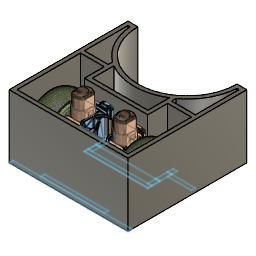
MiniSoccer (Autodesk Fusion 360 design; units mm, degrees)
part number: 2025-12-04-09-52-39-113
Autodesk Fusion 360 part; units mm, degrees
sketch "Sketch1" plane through (0, 0, 0) normal (0, 0, 1) x (1, 0, 0)
  line L0 (0, 0) -> (150, 0)
  line L1 (150, 0) -> (150, -150)
  line L2 (150, -150) -> (0, -150)
  line L3 (0, -150) -> (0, 0)
  line L4 (0, -150) -> (60, -150)
  line L5 (60, -150) -> (60, 0)
  line L6 (60, 0) -> (0, 0)
  line L7 (0, 0) -> (0, -150)
  line L8 (150, -150) -> (90, -150)
  line L9 (90, -150) -> (90, 0)
  line L10 (90, 0) -> (150, 0)
  line L11 (150, 0) -> (150, -150)
  line L12 (0, -150) -> (150, -150)
  line L13 (150, -150) -> (150, -70)
  line L14 (150, -70) -> (0, -70)
  line L15 (0, -70) -> (0, -150)
  line L16 (0, -75) -> (150, -75)
  line L17 (75, -150) -> (75, 0)
  line L18 (75, -70) -> (73.1201, -70)
  line L19 (75, 0) -> (75, -35)
  line L20 (125, -70) -> (25, -70)
  line L21 (25, -70) -> (25, 0)
  line L22 (25, 0) -> (125, 0)
  line L23 (125, 0) -> (125, -70)
  line L24 (35, -70) -> (115, -70)
  line L25 (115, -70) -> (115, -150)
  line L26 (115, -150) -> (35, -150)
  line L27 (35, -150) -> (35, -70)
  line L28 (55, -150) -> (55, -70)
  line L29 (95, -150) -> (95, -70)
  arc A0 (5, 0) -> (145, 0) centre (75, 0) ccw
  line L30 (5, 0) -> (5, -70)
  line L31 (145, 0) -> (145, -3.358)
  line L32 (145, -3.358) -> (145, -70)
  arc A1 (15, 0) -> (135, 0) centre (75, 0) ccw
  arc A2 (10, 0) -> (140, 0) centre (75, 0) ccw
  line L33 (35, -70) -> (35, -44.7214)
  line L34 (115, -70) -> (115, -44.7214)
  line L35 (150, -150) -> (146, -150)
  line L36 (146, -150) -> (146, -75)
  line L37 (146, -75) -> (150, -75)
  line L38 (150, -75) -> (150, -150)
  line L39 (0, -75) -> (4, -75)
  line L40 (4, -75) -> (4, -150)
  line L41 (4, -150) -> (0, -150)
  line L42 (0, -150) -> (0, -75)
  line L43 (150, -150) -> (0, -150)
  line L44 (0, -150) -> (0, -146)
  line L45 (0, -146) -> (150, -146)
  line L46 (150, -146) -> (150, -150)
  line L47 (150, 0) -> (0, 0)
  line L48 (0, 0) -> (0, -5)
  line L49 (0, -5) -> (150, -5)
  line L50 (150, -5) -> (150, 0)
  line L51 (130, -5) -> (145, -5)
  line L52 (145, -5) -> (145, -25)
  line L53 (145, -25) -> (130, -25)
  line L54 (130, -25) -> (130, -5)
  line L55 (20, -5) -> (5, -5)
  line L56 (5, -5) -> (5, -25)
  line L57 (5, -25) -> (20, -25)
  line L58 (20, -25) -> (20, -5)
  point P0 (75, -35)
  dimension "d1" = 150
  dimension "d2" = 150
  dimension "d3" = 60
  dimension "d4" = 150
  dimension "d5" = 60
  dimension "d6" = 80
  dimension "d7" = 100
  dimension "d8" = 70
  constraint horizontal L0
  constraint vertical L1
  constraint horizontal L2
  constraint vertical L3
  constraint coincident L0.start L3.end
  constraint horizontal L4
  constraint vertical L5
  constraint horizontal L6
  constraint vertical L7
  constraint horizontal L8
  constraint vertical L9
  constraint horizontal L10
  constraint vertical L11
  constraint horizontal L12
  constraint vertical L13
  constraint horizontal L14
  constraint vertical L15
  constraint midpoint L3 L16.start
  constraint midpoint L1 L16.end
  constraint midpoint L12 L17.start
  constraint midpoint L0 L17.end
  constraint perpendicular L0 L17
  constraint midpoint L14 L18.start
  constraint coincident L14 L18.end
  constraint coincident L17 P0
  constraint horizontal L20
  constraint perpendicular L20 L21
  constraint parallel L20 L22
  constraint parallel L21 L23
  constraint coincident P0 L19.end
  constraint horizontal L24
  constraint vertical L25
  constraint horizontal L26
  constraint vertical L27
  constraint coincident L8 L25.end
  constraint coincident L14 L24.start
  constraint coincident L4 L28.start
  constraint coincident L14 L28.end
  constraint coincident L24 L29.end
  constraint coincident L17.end L19.start
  constraint coincident L18.start A0
  constraint coincident L0 A0.end
  constraint coincident L0 A0.start
  constraint coincident L14 L30.end
  constraint tangent A0 L30
  constraint tangent A0 L31
  constraint coincident L14 L32.end
  constraint perpendicular L14 L32
  constraint coincident L0 A1.end
  constraint coincident L0 A1.start
  constraint coincident L0 A2.end
  constraint coincident L0 A2.start
  constraint coincident A1 L33.end
  constraint perpendicular L24 L33
  constraint coincident A1 L34.end
  constraint perpendicular L24 L34
  constraint horizontal L35
  constraint vertical L36
  constraint horizontal L37
  constraint vertical L38
  constraint coincident L16 L36.end
  constraint horizontal L39
  constraint vertical L40
  constraint horizontal L41
  constraint vertical L42
  constraint coincident L12 L40.end
  constraint horizontal L43
  constraint vertical L44
  constraint horizontal L45
  constraint vertical L46
  constraint coincident L42 L44.end
  constraint horizontal L47
  constraint vertical L48
  constraint horizontal L49
  constraint vertical L50
  constraint coincident L7 L48.end
  constraint horizontal L51
  constraint vertical L52
  constraint horizontal L53
  constraint vertical L54
  constraint coincident L32 L52.end
  constraint coincident L49 L51.start
  constraint horizontal L55
  constraint vertical L56
  constraint horizontal L57
  constraint vertical L58
  constraint coincident L30 L56.end
  constraint coincident L49 L55.start
  measures "d1" distance of L0.start L0.end
  measures "d2" distance of L0.start L2.end
  measures "d3" distance of L2.end L4.end
  measures "d4" distance of L2.end L0.start
  measures "d5" distance of L1.end L8.end
  measures "d6" distance of L2.end L14.end
  measures "d7" distance of L21.end L22.end
  measures "d8" distance of L20.end L21.end
other "Base Mesh Feature1"
other "Base Mesh Feature2"
other "Modify1"
other "Modify2"
other "Modify3"
other "Modify4"
other "Modify5"
other "Modify6"
other "Modify7"
other "Modify8"
other "Modify9"
other "Modify10"
other "CopyPasteMeshes1"
other "CopyPasteMeshes2"
other "Modify11"
other "Modify12"
other "Modify13"
extrude "Extrude14" cut sketch "Sketch1" along normal blind 60 contours A0 L30 L49 L55 | A0 L30 L49 L55 L56 L57 | L14 L21 A0 L30 L57 | L14 L20 L21 A0 L33 | L5 L14 L20 L24 A0 L33 | L9 L14 L20 L24 A0 L34 | L14 L20 L23 A0 L34 | L14 L23 A0 L32 L53 | A0 L31 L32 L49 L51 | A0 L32 L49 L51 L52 L53
extrude "Extrude16" cut sketch "Sketch1" along normal blind 60 contours L0 L6 A0 A2 L47 L49 L55 | A0 A2 L49 L55 L57 | L21 A0 A2 L57 | L0 L10 A0 A2 L47 L49 L51 | L23 A0 A2 L53 | A0 A2 L49 L51 L53
extrude "Extrude17" cut sketch "Sketch1" along normal blind 60 contours L5 L14 L18 L20 L24 A0 | L5 L17 A0 A2 | L9 L14 L20 L24 A0 | L9 L17 A0 A2
sketch "Sketch2" plane through (0, 0, 0) normal (0, 0, 1) x (1, 0, 0)
  line L0 (150, 0) -> (150, -150)
  line L1 (150, -150) -> (0, -150)
  line L2 (0, -150) -> (0, 0)
  line L3 (0, -75) -> (150, -75)
  line L4 (145, -145) -> (5, -145)
  line L5 (5, -145) -> (5, -5)
  line L6 (145, -5) -> (145, -145)
  line L7 (35, -150) -> (60, -150)
  line L8 (90, -150) -> (115, -150)
  line L9 (90, -50) -> (90, -150)
  line L10 (35, -145) -> (5, -145)
  line L11 (5, -145) -> (5, -65)
  line L12 (5, -65) -> (35, -65)
  line L13 (35, -65) -> (35, -145)
  line L14 (145, -145) -> (115, -145)
  line L15 (115, -145) -> (115, -65)
  line L16 (115, -65) -> (145, -65)
  line L17 (145, -65) -> (145, -145)
  line L18 (5, -105) -> (35, -105)
  line L19 (115, -105) -> (145, -105)
  line L20 (130, -65) -> (130, -145)
  line L21 (20, -65) -> (20, -145)
  arc A0 (12.5, 0) -> (137.5, 0) centre (75, 0) ccw
  line L22 (137.5, -50) -> (12.5, -50)
  line L23 (12.5, -50) -> (12.5, 0)
  line L24 (137.5, 0) -> (137.5, -50)
  arc A1 (7.5, 0) -> (142.5, 0) centre (75, 0) ccw
  line L25 (0, 0) -> (12.5, 0)
  line L26 (5, -5) -> (12.7003, -5)
  line L27 (35, -48.0234) -> (35, -150)
  line L28 (60, -150) -> (60, -50)
  line L29 (75, -50) -> (75, -150)
  line L30 (137.5, -50) -> (123.8043, -39.0434) construction
  line L31 (115, -150) -> (115, -48.0234)
  line L32 (115, -5) -> (115, 0)
  line L33 (137.2997, -5) -> (145, -5)
  line L34 (137.5, 0) -> (150, 0)
  line L35 (14.1146, -14.1146) -> (5, -5) construction
  line L36 (12.5, -50) -> (26.1957, -39.0434) construction
  line L37 (145, -145) -> (50, -50) construction
  line L38 (5, -145) -> (75, -75) construction
  line L39 (82.9725, -67.0275) -> (100, -50) construction
  line L40 (135.8854, -14.1146) -> (145, -5) construction
  point P0 (75, 0)
  dimension "d55" = 125
  constraint horizontal L25
  constraint vertical L0
  constraint horizontal L1
  constraint vertical L2
  constraint coincident L2.end L25.start
  constraint midpoint L2 L3.start
  constraint midpoint L0 L3.end
  constraint midpoint L1 L29.end
  constraint horizontal L4
  constraint perpendicular L4 L5
  constraint parallel L4 L26
  constraint parallel L5 L6
  constraint coincident L38.end L37
  constraint midpoint L3 L38.end
  constraint horizontal L7
  constraint vertical L28
  constraint coincident L1 L7.start
  constraint horizontal L8
  constraint vertical L31
  constraint vertical L9
  constraint coincident L32.end L25
  constraint coincident L1 L8.start
  constraint horizontal L10
  constraint vertical L11
  constraint horizontal L12
  constraint vertical L13
  constraint coincident L5 L11.end
  constraint coincident L4 L10.start
  constraint horizontal L14
  constraint vertical L15
  constraint horizontal L16
  constraint vertical L17
  constraint coincident L15.end L31
  constraint midpoint L11 L18.start
  constraint midpoint L13 L18.end
  constraint midpoint L15 L19.start
  constraint midpoint L17 L19.end
  constraint midpoint L16 L20.start
  constraint midpoint L14 L20.end
  constraint midpoint L12 L21.start
  constraint midpoint L10 L21.end
  constraint coincident A0.end L25
  constraint horizontal L22
  constraint perpendicular L22 L23
  constraint coincident P0 L30
  constraint coincident P0 L36
  constraint coincident A1.start L25
  constraint coincident A1.end L25
  constraint coincident A0 L26.end
  constraint coincident L22 L29.start
  constraint collinear L31 L32
  constraint coincident A0 L33.start
  constraint coincident L22 L28.end
  constraint coincident L22 L9.start
  constraint coincident A0 L35.start
  constraint collinear L35 L37
  constraint coincident A0 L36.end
  constraint coincident L22 L37.end
  constraint coincident A0 L27.start
  constraint coincident A1 L39.start
  constraint collinear L38 L39
  constraint coincident L22 L39.end
  constraint coincident A0 L40.start
  constraint coincident A0 L31.end
  constraint coincident A0 L30.end
  measures "d55" diameter of A0
other "Modify14"
other "Modify15"
extrude "Extrude24" add sketch "Sketch2" along normal blind 80 separate body contours L0 L3 L6 L17 A1 L33 L34 | L0 L1 L3 L4 L6 L14 L17 L31 | L24 A1 L33 L34 | L1 L4 L8 L9 L31 | L1 L4 L9 L29 | L1 L4 L28 L29 | L1 L4 L7 L27 L28 | L1 L2 L3 L4 L5 L10 L11 L27 | L2 L3 L5 L11 A1 L25 L26 | L23 A1 L25 L26 makes body 1
other "Modify16"
other "Modify17"
other "Modify18"
other "Modify19"
other "CopyPasteMeshes3"
other "Modify20"
other "Modify21"
extrude "Extrude25" add sketch "Sketch2" along normal blind 80 contours L24 A1 L33 | A0 L22 L24 A1 L31 L33 | L22 A1 L31 | A0 L22 L31 | L9 A0 L22 A1 L31 | L9 A0 A1 L29 | A0 A1 L28 L29 | A0 L22 A1 L27 L28 | L22 A1 L27 | A0 L22 L27 | A0 L22 L23 A1 L26 L27 | L23 A1 L26 bodies 1
other "Base Mesh Feature3"
other "Modify22"
other "Modify23"
other "Modify24"
other "Modify25"
other "Modify26"
other "Modify27"
sketch "Sketch3" plane through (0, 0, 0) normal (0, 0, 1) x (1, 0, 0)
  line L0 (35, -75) -> (115, -75)
  line L1 (115, -75) -> (115, -90)
  line L2 (115, -90) -> (35, -90)
  line L3 (35, -90) -> (35, -75)
  line L4 (35, -90) -> (115, -90)
  line L5 (115, -90) -> (115, -85)
  line L6 (115, -85) -> (35, -85)
  line L7 (35, -85) -> (35, -90)
  line L8 (35, -145) -> (115, -145)
  line L9 (115, -145) -> (115, -140)
  line L10 (115, -140) -> (35, -140)
  line L11 (35, -140) -> (35, -145)
  line L12 (0, -145) -> (150, -145)
  line L13 (150, -145) -> (150, -150)
  line L14 (150, -150) -> (0, -150)
  line L15 (0, -150) -> (0, -145)
  line L16 (110, -75) -> (115, -75)
  line L17 (115, -75) -> (115, -60)
  line L18 (115, -60) -> (110, -60)
  line L19 (110, -60) -> (110, -75)
  line L20 (145, -65) -> (115, -65)
  line L21 (115, -65) -> (115, -60)
  line L22 (115, -60) -> (145, -60)
  line L23 (145, -60) -> (145, -65)
  line L24 (35, -75) -> (40, -75)
  line L25 (40, -75) -> (40, -60)
  line L26 (40, -60) -> (35, -60)
  line L27 (35, -60) -> (35, -75)
  line L28 (35, -60) -> (5, -60)
  line L29 (5, -60) -> (5, -65)
  line L30 (5, -65) -> (35, -65)
  line L31 (35, -65) -> (35, -60)
  line L32 (35, -60) -> (40, -60)
  line L33 (40, -60) -> (40, -54.3331)
  line L34 (40, -54.3331) -> (35, -54.3331)
  line L35 (35, -54.3331) -> (35, -60)
  line L36 (110, -60) -> (115, -60)
  line L37 (115, -60) -> (115, -53.1436)
  line L38 (115, -53.1436) -> (110, -53.1436)
  line L39 (110, -53.1436) -> (110, -60)
  line L40 (35, -75) -> (40, -75)
  line L41 (40, -75) -> (40, -85)
  line L42 (40, -85) -> (35, -85)
  line L43 (35, -85) -> (35, -75)
  line L44 (110, -75) -> (115, -75)
  line L45 (115, -75) -> (115, -85)
  line L46 (115, -85) -> (110, -85)
  line L47 (110, -85) -> (110, -75)
  constraint horizontal L0
  constraint vertical L1
  constraint horizontal L2
  constraint vertical L3
  constraint horizontal L4
  constraint vertical L5
  constraint horizontal L6
  constraint vertical L7
  constraint coincident L1 L5.end
  constraint horizontal L8
  constraint vertical L9
  constraint horizontal L10
  constraint vertical L11
  constraint horizontal L12
  constraint vertical L13
  constraint horizontal L14
  constraint vertical L15
  constraint horizontal L16
  constraint vertical L17
  constraint horizontal L18
  constraint vertical L19
  constraint coincident L0 L16.start
  constraint horizontal L20
  constraint vertical L21
  constraint horizontal L22
  constraint vertical L23
  constraint horizontal L24
  constraint vertical L25
  constraint horizontal L26
  constraint vertical L27
  constraint horizontal L28
  constraint vertical L29
  constraint horizontal L30
  constraint vertical L31
  constraint horizontal L32
  constraint vertical L33
  constraint horizontal L34
  constraint vertical L35
  constraint horizontal L36
  constraint vertical L37
  constraint horizontal L38
  constraint vertical L39
  constraint horizontal L40
  constraint vertical L41
  constraint horizontal L42
  constraint vertical L43
  constraint coincident L6 L41.end
  constraint horizontal L44
  constraint vertical L45
  constraint horizontal L46
  constraint vertical L47
extrude "Extrude26" add sketch "Sketch3" along normal blind 80 separate body contours L1 L2 L3 L4 L5 L6 L7 L42 L46 makes body 2
extrude "Extrude27" add sketch "Sketch2" along normal blind 5 contours L3 L4 L9 L15 L31 | L3 L4 L9 L29 | L3 L4 L28 L29 | L3 L4 L13 L27 L28 bodies 2
extrude "Extrude28" add sketch "Sketch2" along normal blind 5 contours L6 L16 L22 L24 A1 L31 L33 | L22 L24 A1 | L3 L9 L15 A1 L31 | L3 L9 A1 L29 | L3 A1 L28 L29 | L3 L13 A1 L27 L28 | L5 L12 L22 L23 A1 L26 L27 | L22 L23 A1 bodies 1 2
extrude "Extrude29" cut sketch "Sketch3" along normal blind 80 contours L8 L12 L13 L14 L15 bodies 1
extrude "Extrude30" add sketch "Sketch3" along normal blind 80 contours L0 L24 L25 L26 L27 L31 L32 L40 | L27 L28 L29 L30 L31 | L0 L16 L17 L18 L19 L21 L36 L44 | L17 L20 L21 L22 L23 bodies 1
extrude "Extrude31" add sketch "Sketch2" along normal blind 80 contours A0 L24 L33 bodies 1
extrude "Extrude32" add sketch "Sketch2" along normal blind 80 contours A0 L23 L26 bodies 1
other "Base Mesh Feature4"
other "Modify28"
other "Modify29"
extrude "Extrude33" add sketch "Sketch3" along normal blind 80 contours L8 L12 L13 L14 L15 bodies 1
extrude "Extrude34" cut sketch "Sketch2" along normal blind 5 contours L6 L16 L22 L24 A1 L31 L33 | L22 L24 A1 | L5 L12 L22 L23 A1 L26 L27 | L22 L23 A1 bodies 1
extrude "Extrude35" add sketch "Sketch3" along normal blind 5 contours L27 L28 L29 L30 L31 | L17 L20 L21 L22 L23 bodies 1
extrude "Extrude36" add sketch "Sketch3" along normal blind 80 contours L0 L3 L6 L24 L40 L41 L42 L43 | L0 L1 L6 L16 L44 L45 L46 L47 | L26 L32 L33 L34 L35 | L18 L36 L37 L38 L39 bodies 1
sketch "Sketch4" plane through (0, -90, 0) normal (0, -1, 0) x (1, 0, 0)
  line L0 (35, 5) -> (115, 5)
  line L1 (115, 5) -> (115, 80)
  line L2 (115, 80) -> (35, 80)
  line L3 (35, 80) -> (35, 5)
  line L4 (65, 15) -> (84, 15)
  line L5 (84, 15) -> (84, 52)
  line L6 (84, 52) -> (65, 52)
  line L7 (65, 52) -> (65, 15)
  constraint horizontal L4
  constraint vertical L5
  constraint horizontal L6
  constraint vertical L7
other "Modify30"
extrude "Extrude37" cut sketch "Sketch4" against normal blind 5 contours L4 L5 L6 L7 bodies 1
